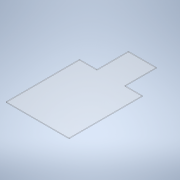
# Autodesk Inventor part: Lexan Underbelly
Saved by Autodesk Inventor 2021 (Build 250183000, 183)
## iProperties
Created: 2021-03-06
Part Number: Lexan Underbelly
Material: Polycarbonate, Clear
Document SubType Name: Modeling
Designer: aidan
Density: 1.2 g/cm^3
Appearance: Polycarbonate - Clear
Author: aidan
Autodesk Inventor part; units mm, degrees
ref_plane "YZ Plane" through (0, 0, 0) normal (1, 0, 0) x (0, 1, 0)
ref_plane "XZ Plane" through (0, 0, 0) normal (0, 1, 0) x (-1, 0, 0)
ref_plane "XY Plane" through (0, 0, 0) normal (0, 0, 1) x (1, 0, 0)
sketch "Sketch1" plane through (0, 0, 0) normal (0, 1, 0) x (-1, 0, 0)
  line L0 (0, 0) -> (0, -533.4)
  line L1 (0, -533.4) -> (-127, -533.4)
  line L2 (-127, -533.4) -> (-127, -762)
  line L3 (-127, -762) -> (-330.2, -762)
  line L4 (-330.2, -762) -> (-330.2, -533.4)
  line L5 (-330.2, -533.4) -> (-457.2, -533.4)
  line L6 (-457.2, -533.4) -> (-457.2, 0)
  line L7 (-457.2, 0) -> (0, 0)
  point P0 (-127, -647.7)
  point P1 (-330.2, -647.7)
  dimension "d0" = 203.2
  dimension "d1" = 228.6
  dimension "d2" = 127
  dimension "d3" = 533.4
  constraints: 16 end point, 3 perpendicular, 3 vertical, 2 midpoint, 2 parallel, 1 collinear, 1 point on line
  measures "d0" distance of L2.end L3.end
  measures "d1" distance of L3.end L4.end
  measures "d2" distance of L4.end L5.end
  measures "d3" distance of L5.end L6.end
extrude "Extrusion1" add sketch "Sketch1" along normal blind 5.588
body "Solid1"
